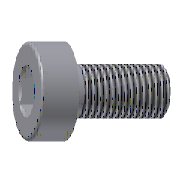
# Autodesk Inventor part: M 8x60
Saved by Autodesk Inventor 2022.2 (Build 262287000, 287)
## iProperties
Created: 2021-02-02
Part Number: M 8x60
Material: Stahl, weich
Description: Inbusschraube DIN 912 - 12.9
Document SubType Name: Modeling
Designer: jan
Standard Revision: 1
Manufacturer: DME
Language: de-DE
Size Designation: 8x60
Categories: <MemberInstance><Categories><Category DisplayName="Werkzeug" InternalName="349578f2-f4d4-4954-8c09-8e99297a61c0" Mnemonic="MOLD"><Category DisplayName="Schraube" InternalName="aa59405f-205a-41d7-8d32-e7f5149a4020" Mnemonic="FASTENERS"><Category DisplayName="Schraube" InternalName="90c4b15c-124d-4e03-b133-f81a19b25973" Mnemonic="BOLTS"><CategoryParameter DisplayName="Nenndurchmesser" InternalName="05a2f57c-ca5a-4d7d-bd85-46c8a217905e" Mnemonic="NOMINAL DIAMETER"/><CategoryParameter DisplayName="Nennlänge" InternalName="14e897c5-944a-4dd6-b303-a06affccee6b" Mnemonic="NOMINAL LENGTH"/><CategoryParameter DisplayName="Gewinde Bezeichnung" InternalName="57520822-b941-44ed-9338-7c3722cf9cad" Mnemonic="THREAD DESIGNATION"/><CategoryParameter DisplayName="Gewinde Richtung" InternalName="7080e064-a078-46ab-901b-aa29ad61c587" Mnemonic="THREAD DIRECTION"/><CategoryParameter DisplayName="Gewinde Familie" InternalName="8447d7ec-7e7a-4c55-9f9e-e7d45a47ca2a" Mnemonic="THREAD TYPE"/><CategoryParameter DisplayName="Gewinde Klasse" InternalName="8464a6bd-02ed-4ee6-a4ba-4f8d953a1c5f" Mnemonic="THREAD CLASS"/><Category DisplayName="Zylinderschraube mit Innensechskant" InternalName="dec64631-5a3f-4cf9-a54d-52cede3536d0" Mnemonic="SOCKET HEAD CAP SCREWS"><CategoryParameter DisplayName="Gewindelänge" InternalName="4ed31c41-e890-460b-a17d-04acefc35541" Mnemonic="THREAD LENGTH"/><CategoryParameter DisplayName="Kopfdurchmesser" InternalName="510cdbb5-2cc6-4f20-b042-c04fe0ff78fc" Mnemonic="HEAD DIAMETER"/><CategoryParameter DisplayName="Kopfhöhe" InternalName="851bf056-7b30-4dcc-aa43-a86407258e2a" Mnemonic="HEAD HEIGHT"/></Category></Category></Category></Category><Category DisplayName="Datentyp" InternalName="23b78d0f-2648-40c6-8793-ca6db495c9e8" Mnemonic="DATATYPE"><CategoryParameter DisplayName="Anzeigename" InternalName="05415f3d-3907-474b-a020-eb9d644f4cf3" Mnemonic="DISPLAYNAME"/><CategoryParameter DisplayName="Norm" InternalName="0c0a119c-1e12-4c84-803f-101930972f5e" Mnemonic="STANDARD"/><CategoryParameter DisplayName="Beschreibung" InternalName="13903e3d-64b1-4950-80da-f627842ea37f" Mnemonic="DESCRIPTION"/><CategoryParameter DisplayName="Bezeichnung" InternalName="2675968c-4ce5-49e0-a4f5-552d29089031" Mnemonic="DESIGNATION"/><CategoryParameter DisplayName="Standardzeile" InternalName="2af9ec52-faaa-4026-b378-f9fa4afca842" Mnemonic="DEFAULTROW"/><CategoryParameter DisplayName="Ordnername" InternalName="3f06958e-8713-4116-9be7-ed6184ecc97b" Mnemonic="FOLDERNAME"/><CategoryParameter DisplayName="Revisionsanleitung" InternalName="45a75005-10b1-4dfc-8d6d-dfe629f0b93c" Mnemonic="REVISIONGUID"/><CategoryParameter DisplayName="Dateiname" InternalName="8b46a4cc-9585-4fed-90c3-899f57e09a73" Mnemonic="FILENAME"/><CategoryParameter DisplayName="Normungsorganisation" InternalName="8f5914e1-4693-403f-8ab5-d37768198c9d" Mnemonic="STDSORG"/><CategoryParameter DisplayName="Gruppenversion" InternalName="914462f6-6e19-4b14-ba84-155b9680b1d0" Mnemonic="FAMILYREVISION"/><CategoryParameter DisplayName="Normrevision" InternalName="91d5a463-65c2-4fde-b823-3b7fea5e8e17" Mnemonic="STANDARDREVISION"/><CategoryParameter DisplayName="Variantenrevision" InternalName="a65d44b9-392f-4f4f-857b-e4b3d54996fe" Mnemonic="MEMBERREVISION"/><CategoryParameter DisplayName="ClipFormat" InternalName="bc51e27b-3422-4e78-93ef-cec197ddf230" Mnemonic="CLIPFORMAT"/><CategoryParameter DisplayName="Hersteller" InternalName="cd6c7a72-a28a-4e50-99a9-2c7f4e13e5ad" Mnemonic="MANUFACTURER"/><CategoryParameter DisplayName="InternerName" InternalName="cf1d0246-76d9-4b4a-8305-fa0409afb5c1" Mnemonic="INTERNALNAME"/><CategoryParameter DisplayName="IstMetrisch" InternalName="e2385c5b-1ea4-4823-96a8-8de651266ec3" Mnemonic="ISMETRIC"/><Category DisplayName="Bauteil" InternalName="c0e0b642-3bcb-4cc8-9e80-f96d35c4afa4" Mnemonic="PART"><CategoryParameter DisplayName="Bauteilnummer" InternalName="016b6077-bfbe-49bd-92c9-d8d59c39c941" Mnemonic="PARTNUMBER"/><CategoryParameter DisplayName="Bestandsnummer" InternalName="4dba7c1c-e26c-444e-836c-b08b433409a8" Mnemonic="STOCKNUMBER"/><CategoryParameter DisplayName="Materialschlüssel" InternalName="5c9a8adb-dd2b-4535-b97f-0a94a95fe41f" Mnemonic="MATERIALKEY"/><CategoryParameter DisplayName="Material" InternalName="818a152a-d3c3-49ca-80ee-df7d91421b8e" Mnemonic="MATERIAL"/></Category></Category></Categories><FamilyTemplate Id="M"><FamilyTemplateParameters><FamilyTemplateParameter ObjectType="kUserParameterObject" ValueType="xs:double" Id="1" ObjectReferenceKey="d"/><FamilyTemplateParameter ObjectType="kUserParameterObject" ValueType="xs:double" Id="2" ObjectReferenceKey="L"/><FamilyTemplateParameter ObjectType="kUserParameterObject" ValueType="xs:double" Id="3" ObjectReferenceKey="dk"/><FamilyTemplateParameter ObjectType="kUserParameterObject" ValueType="xs:double" Id="4" ObjectReferenceKey="b"/><FamilyTemplateParameter ObjectType="kUserParameterObject" ValueType="xs:double" Id="5" ObjectReferenceKey="k"/><FamilyTemplateParameter ObjectType="kUserParameterObject" ValueType="xs:double" Id="6" ObjectReferenceKey="sw"/><FamilyTemplateParameter ObjectType="kUserParameterObject" ValueType="xs:double" Id="7" ObjectReferenceKey="t"/><FamilyTemplateParameter ObjectType="kUserParameterObject" ValueType="xs:double" Id="8" ObjectReferenceKey="P"/><FamilyTemplateParameter ObjectType="kThreadFeatureObject" ValueType="xs:string" Id="9" ObjectReferenceKey="1002000010000000e9590000000000008000000000000000" SubObjectId="ThreadInfo"><FamilyTemplateParameter ObjectType="" ValueType="xs:string" Id="10" SubObjectId="ThreadType"/><FamilyTemplateParameter ObjectType="" ValueType="xs:string" Id="11" SubObjectId="ThreadDesignation"/><FamilyTemplateParameter ObjectType="" ValueType="xs:string" Id="12" SubObjectId="ThreadClass"/><FamilyTemplateParameter ObjectType="" ValueType="xs:string" Id="13" SubObjectId="ThreadDirection"/></FamilyTemplateParameter><FamilyTemplateParameter ObjectType="kPartComponentDefinitionObject" ValueType="xs:string" Id="14" SubObjectId="Material"/><FamilyTemplateParameter ObjectType="kPropertyObject" ValueType="xs:string" Id="23" ObjectReferenceKey="{32853F0F-3444-11d1-9E93-0060B03C1CA6}" SubObjectId="5"/><FamilyTemplateParameter ObjectType="kPropertyObject" ValueType="xs:string" Id="24" ObjectReferenceKey="{32853F0F-3444-11d1-9E93-0060B03C1CA6}" SubObjectId="52"/></FamilyTemplateParameters></FamilyTemplate><CategoryParameterMap><ParamToTemplateMap><ParamToTemplate CategoryParameter="//CategoryParameter[@InternalName='2af9ec52-faaa-4026-b378-f9fa4afca842']" ConstantValue="1"/><ParamToTemplate CategoryParameter="//CategoryParameter[@InternalName='bc51e27b-3422-4e78-93ef-cec197ddf230']" ConstantValue="CF_INVENTOR.STDPARTS"/><ParamToTemplate CategoryParameter="//CategoryParameter[@InternalName='e2385c5b-1ea4-4823-96a8-8de651266ec3']" ConstantValue="true"/><ParamToTemplate CategoryParameter="//CategoryParameter[@InternalName='cf1d0246-76d9-4b4a-8305-fa0409afb5c1']" ConstantValue="004b52fc-a597-4a52-971e-5f4d7a0fb02e"/><ParamToTemplate CategoryParameter="//CategoryParameter[@InternalName='45a75005-10b1-4dfc-8d6d-dfe629f0b93c']" ConstantValue="bf5d47f6-4819-43f5-b2be-980df9fc057f"/><ParamToTemplate CategoryParameter="//CategoryParameter[@InternalName='3f06958e-8713-4116-9be7-ed6184ecc97b']" ConstantValue="M"/><ParamToTemplate CategoryParameter="//CategoryParameter[@InternalName='8f5914e1-4693-403f-8ab5-d37768198c9d']" TemplateParameter="18"/><ParamToTemplate CategoryParameter="//CategoryParameter[@InternalName='0c0a119c-1e12-4c84-803f-101930972f5e']" TemplateParameter="19"/><ParamToTemplate CategoryParameter="//CategoryParameter[@InternalName='91d5a463-65c2-4fde-b823-3b7fea5e8e17']" ConstantValue="1"/><ParamToTemplate CategoryParameter="//CategoryParameter[@InternalName='cd6c7a72-a28a-4e50-99a9-2c7f4e13e5ad']" ConstantValue="DME"/><ParamToTemplate CategoryParameter="//CategoryParameter[@InternalName='13903e3d-64b1-4950-80da-f627842ea37f']" ConstantValue="Socket Head Cap Screw DIN 912 - 12.9"/><ParamToTemplate CategoryParameter="//CategoryParameter[@InternalName='05415f3d-3907-474b-a020-eb9d644f4cf3']" ConstantValue="M"/><ParamToTemplate CategoryParameter="//CategoryParameter[@InternalName='914462f6-6e19-4b14-ba84-155b9680b1d0']" ConstantValue="1"/><ParamToTemplate CategoryParameter="//CategoryParameter[@InternalName='bc51e27b-3422-4e78-93ef-cec197ddf230']" ConstantValue="CF_INVENTOR.STDPARTS"/><ParamToTemplate CategoryParameter="//CategoryParameter[@InternalName='8b46a4cc-9585-4fed-90c3-899f57e09a73']" ConstantValue="M 8x60"/><ParamToTemplate CategoryParameter="//CategoryParameter[@InternalName='a65d44b9-392f-4f4f-857b-e4b3d54996fe']" ConstantValue="5A7904A5-9283-41B0-8AEC-383EFFE79F07"/><ParamToTemplate CategoryParameter="//CategoryParameter[@InternalName='2675968c-4ce5-49e0-a4f5-552d29089031']" TemplateParameter="24"/><ParamToTemplate CategoryParameter="//CategoryParameter[@InternalName='14e897c5-944a-4dd6-b303-a06affccee6b']" TemplateParameter="2"/><ParamToTemplate CategoryParameter="//CategoryParameter[@InternalName='818a152a-d3c3-49ca-80ee-df7d91421b8e']" TemplateParameter="14"/><ParamToTemplate CategoryParameter="//CategoryParameter[@InternalName='016b6077-bfbe-49bd-92c9-d8d59c39c941']" TemplateParameter="23"/><ParamToTemplate CategoryParameter="//CategoryParameter[@InternalName='8464a6bd-02ed-4ee6-a4ba-4f8d953a1c5f']" TemplateParameter="12"/><ParamToTemplate CategoryParameter="//CategoryParameter[@InternalName='57520822-b941-44ed-9338-7c3722cf9cad']" TemplateParameter="11"/><ParamToTemplate CategoryParameter="//CategoryParameter[@InternalName='7080e064-a078-46ab-901b-aa29ad61c587']" TemplateParameter="13"/><ParamToTemplate CategoryParameter="//CategoryParameter[@InternalName='8447d7ec-7e7a-4c55-9f9e-e7d45a47ca2a']" TemplateParameter="10"/><ParamToTemplate CategoryParameter="//CategoryParameter[@InternalName='4ed31c41-e890-460b-a17d-04acefc35541']" TemplateParameter="4"/><ParamToTemplate CategoryParameter="//CategoryParameter[@InternalName='05a2f57c-ca5a-4d7d-bd85-46c8a217905e']" TemplateParameter="1"/><ParamToTemplate CategoryParameter="//CategoryParameter[@InternalName='510cdbb5-2cc6-4f20-b042-c04fe0ff78fc']" TemplateParameter="3"/><ParamToTemplate CategoryParameter="//CategoryParameter[@InternalName='851bf056-7b30-4dcc-aa43-a86407258e2a']" TemplateParameter="5"/></ParamToTemplateMap></CategoryParameterMap></MemberInstance>
Mass: 30.828 g
Surface Area: 21.6203 cm^2
Volume: 3.92714 cm^3
Density: 7.85 g/cm^3
Appearance: Halbpoliert
IsCustomPart: 0
Author: jan
Autodesk Inventor part; units mm, degrees
ref_plane "YZ Plane" through (0, 0, 0) normal (1, 0, 0) x (0, 1, 0)
ref_plane "XZ Plane" through (0, 0, 0) normal (0, 1, 0) x (-1, 0, 0)
ref_plane "XY Plane" through (0, 0, 0) normal (0, 0, 1) x (1, 0, 0)
sketch "Sketch1" plane through (0, 0, 0) normal (1, 0, 0) x (0, 1, 0)
  line L0 (0, -73.6) -> (0, 21.6) projected
  line L1 (3.4641, 8) -> (6.5, 8)
  line L2 (6.5, 8) -> (6.5, 0)
  line L3 (6.5, 0) -> (4, 0)
  line L4 (4, 0) -> (4, -60)
  line L5 (4, -60) -> (0, -60)
  line L6 (0, 2.1974) -> (0, -60)
  line L7 (0, 2.1974) -> (3, 4)
  line L8 (3, 4) -> (3, 7.5359)
  line L9 (3, 7.5359) -> (3.4641, 8)
  point P0 (0, 0)
  dimension "d0" = 13
  dimension "d1" = 8
  dimension "d2" = 8
  dimension "d3" = 60
  dimension "d4" = 59
  dimension "d5" = 45
  dimension "d6" = 6
  dimension "d7" = 6.9282
  dimension "d8" = 4
  constraints: 18 end point, 4 vertical, 3 horizontal, 2 point on line
  measures "d0" diameter of L2 L0
  measures "d1" distance between parallel lines of L3 L1
  measures "d2" diameter of L4 L0
  measures "d3" distance between parallel lines of L5 L3
  measures "d4" angle of L0 L7
  measures "d5" angle of L0 L9
  measures "d6" diameter of L8 L0
  measures "d7" diameter of L1.start L0
  measures "d8" distance from line of L7.end L1
revolve "Revolution1" add sketch "Sketch1" angle 360 about axis through (0, 0, -10) along (0, 0, 1)
sketch "Sketch2" plane through (0, 0, 8) normal (0, 0, 1) x (1, 0, 0)
  circle A0 centre (0, 0) radius 3.4641 construction
  line L0 (0, 3.4641) -> (3, 1.7321)
  line L1 (3, 1.7321) -> (3, -1.7321)
  line L2 (3, -1.7321) -> (0, -3.4641)
  line L3 (0, -3.4641) -> (-3, -1.7321)
  line L4 (-3, -1.7321) -> (-3, 1.7321)
  line L5 (-3, 1.7321) -> (0, 3.4641)
  constraints: 12 end point, 2 vertical alignment, 1 coincident, 14 other
extrude "Extrusion1" cut sketch "Sketch2" against normal up to surface round surface about axis through (0, 0, 3.0987) along (0, 0, -1) radius 1.5 half angle -59 far side no
thread "Thread1" size "M8x1.25" class "6g" standard "ISO Metric profile" length 22
chamfer "Chamfer1" distance 0.625 angle 45 1 edges at (0, -4, -60)
fillet "Fillet1" radius 0.625 1 edges at (0, -6.5, 8)
equation "\"d0\" = dk"
equation "\"d1\" = k"
equation "\"d2\" = d"
equation "\"d3\" = L"
equation "\"d6\" = sw"
equation "\"d7\" = 1.1547 * sw"
equation "\"d8\" = t"
equation "\"d10\" = b"
equation "\"d12\" = 0.5 * P"
equation "\"d13\" = 0.5 * P"
equation "\"d\" = 8"
equation "\"L\" = 60"
equation "\"dk\" = 13"
equation "\"b\" = 22"
equation "\"k\" = 8"
equation "\"sw\" = 6"
equation "\"t\" = 4"
equation "\"P\" = 1.25"
body "Solid1"
